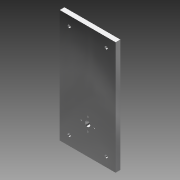
# Autodesk Inventor part: Part74
Saved by Autodesk Inventor 2015 (Build 190159000, 159)
## iProperties
Created: 2015-01-10
Part Number: Part74
Material: Generic
Document SubType Name: Modeling
Designer: mastkee16
Density: 1 g/cm^3
Appearance: Chrome - Polished
Author: mastkee16
Autodesk Inventor part; units mm, degrees
ref_plane "YZ Plane" through (0, 0, 0) normal (1, 0, 0) x (0, 1, 0)
ref_plane "XZ Plane" through (0, 0, 0) normal (0, 1, 0) x (-1, 0, 0)
ref_plane "XY Plane" through (0, 0, 0) normal (0, 0, 1) x (1, 0, 0)
sketch "Sketch1" plane through (0, 0, 0) normal (0, 0, 1) x (1, 0, 0)
  point P0 (0, 0)
sketch "Sketch2" plane through (0, 0, 0) normal (0, 0, 1) x (1, 0, 0)
  line L0 (0, 0) -> (150.622, 0)
  line L1 (150.622, 0) -> (150.622, 304.8)
  line L2 (150.622, 304.8) -> (0, 304.8)
  line L3 (0, 304.8) -> (0, 0)
  circle A0 centre (25.4, 279.4) radius 3.9687
  circle A1 centre (125.222, 279.4) radius 3.9687
  circle A2 centre (25.4, 25.4) radius 3.9688
  circle A3 centre (125.222, 25.4) radius 3.9688
  dimension "d0" = 150.622
  dimension "d1" = 304.8
  dimension "d2" = 7.9375
  dimension "d3" = 25.4
  dimension "d4" = 25.4
  dimension "d5" = 7.9375
  dimension "d6" = 25.4
  dimension "d7" = 25.4
  dimension "d8" = 7.9375
  dimension "d9" = 25.4
  dimension "d10" = 25.4
  dimension "d11" = 7.9375
  dimension "d12" = 25.4
  dimension "d13" = 25.4
  constraints: 8 end point, 4 centre point, 2 parallel, 1 horizontal, 1 perpendicular
  measures "d0" distance of L2.end L1.end
  measures "d1" distance of L1.end L0.end
  measures "d2" diameter of A0
  measures "d3" distance from line of A0.centre L2
  measures "d4" distance from line of L3 A0.centre
  measures "d5" diameter of A1
  measures "d6" distance from line of L1 A1.centre
  measures "d7" distance from line of L2 A1.centre
  measures "d8" diameter of A2
  measures "d9" distance from line of L3 A2.centre
  measures "d10" distance from line of L0 A2.centre
  measures "d11" diameter of A3
  measures "d12" distance from line of L1 A3.centre
  measures "d13" distance from line of L0 A3.centre
extrude "Extrusion1" add sketch "Sketch2" along normal blind 12.7
sketch "Sketch3" plane through (0, 0, 12.7) normal (0, 0, 1) x (1, 0, 0)
  line L0 (150.622, 304.8) -> (0, 304.8) projected
  line L1 (0, 0) -> (150.622, 0) projected
  line L2 (0, 304.8) -> (0, 0) projected
  line L3 (150.622, 0) -> (150.622, 304.8) projected
  circle A0 centre (57.811, 76.2) radius 1.905
  circle A1 centre (75.311, 93.7) radius 1.905
  circle A2 centre (75.311, 58.7) radius 1.905
  circle A3 centre (92.811, 76.2) radius 1.905
  point P0 (75.311, 76.2)
  dimension "d16" = 228.6
  dimension "d17" = 76.2
  dimension "d18" = 75.311
  dimension "d19" = 75.311
  dimension "d31" = 3.81
  dimension "d32" = 3.81
  dimension "d33" = 3.81
  dimension "d34" = 3.81
  dimension "d45" = 34.9999
  dimension "d46" = 17.5
  dimension "d47" = 17.5
  dimension "d48" = 17.5
  constraints: 4 centre point, 4 coincident
  measures "d16" distance from line of point (75.311, 76.2) L0
  measures "d17" distance from line of point (75.311, 76.2) L1
  measures "d18" distance from line of L2 point (75.311, 76.2)
  measures "d19" distance from line of L3 point (75.311, 76.2)
  measures "d31" diameter of A0
  measures "d32" diameter of A1
  measures "d33" diameter of A2
  measures "d34" diameter of A3
  measures "d45" distance of point (75.311, 58.7) point (75.311, 93.7)
  measures "d46" distance of point (75.311, 76.2) point (75.311, 93.7)
  measures "d47" distance of point (75.311, 76.2) point (92.811, 76.2)
  measures "d48" distance of point (75.311, 76.2) point (57.811, 76.2)
hole "Hole1" at (75.311, 76.2, 12.7) direction (0, 0, -1) diameter 13.97 end through all
extrude "Extrusion2" cut sketch "Sketch3" against normal blind 25.4 contours A0 | A1 | A2 | A3
body "Solid1"
